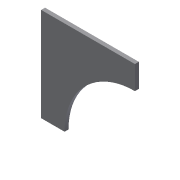
# Autodesk Inventor part: support
Saved by Autodesk Inventor 2022 (Build 260148000, 148)
## iProperties
Created: 2007-01-12
Part Number: support
Document SubType Name: Modeling
Designer: ceirmann
Density: 1 g/cm^3
Material: Generic
Appearance: Default
Author: ceirmann
Autodesk Inventor part; units mm, degrees
ref_plane "YZ Plane" through (0, 0, 0) normal (1, 0, 0) x (0, 1, 0)
ref_plane "XZ Plane" through (0, 0, 0) normal (0, 1, 0) x (-1, 0, 0)
ref_plane "XY Plane" through (0, 0, 0) normal (0, 0, 1) x (1, 0, 0)
sketch "Sketch1" plane through (0, 0, 0) normal (0, 0, 1) x (1, 0, 0)
  line L0 (0, 0) -> (0, -152.4)
  line L1 (0, -152.4) -> (38.1, -152.4)
  arc A0 (152.4, -38.1) -> (38.1, -152.4) centre (152.4, -152.4) ccw
  line L2 (152.4, -38.1) -> (152.4, 0)
  line L3 (152.4, 0) -> (0, 0)
  dimension "d0" = 152.4
  dimension "d1" = 152.4
  dimension "d2" = 38.1
  dimension "d3" = 38.1
  constraints: 8 end point, 2 parallel, 2 point on circle, 1 centre point, 1 perpendicular, 1 point on line, 1 vertical
  measures "d0" distance of L2.end L0.start
  measures "d1" distance of L0.start L0.end
  measures "d2" distance of L2.start L2.end
  measures "d3" distance of L0.end L1.end
extrude "Extrusion1" add sketch "Sketch1" against normal blind 6.35
body "Solid1"
